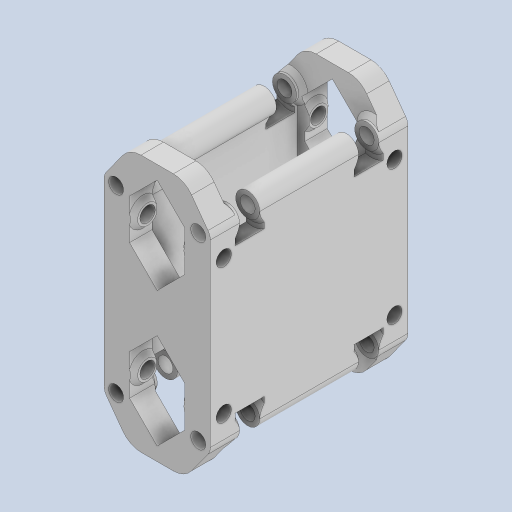
# Autodesk Inventor part: 3d_slider
Saved by Autodesk Inventor 2024 (Build 280153000, 153)
## iProperties
Created: 2023-08-10
Part Number: 3d_slider
Material: 一般
Document SubType Name: Modeling
Designer: zegi
Density: 1 g/cm^3
Appearance: 既定
Author: zegi
Autodesk Inventor part; units mm, degrees
ref_plane "YZ Plane" through (0, 0, 0) normal (1, 0, 0) x (0, 1, 0)
ref_plane "XZ Plane" through (0, 0, 0) normal (0, 1, 0) x (-1, 0, 0)
ref_plane "XY Plane" through (0, 0, 0) normal (0, 0, 1) x (1, 0, 0)
sketch "スケッチ1" plane through (0, 0, 0) normal (0, 0, 1) x (1, 0, 0)
  line L0 (-5.15, -39.6311) -> (5.15, -39.6311)
  line L1 (5.15, -39.6311) -> (5.15, 39.6311)
  line L2 (5.15, 39.6311) -> (-5.15, 39.6311)
  line L3 (-5.15, 39.6311) -> (-5.15, -39.6311)
  line L4 (-5.15, -39.6311) -> (5.15, 39.6311) construction
  line L5 (5.15, -39.6311) -> (-5.15, 39.6311) construction
  circle A0 centre (9.15, 20) radius 4 construction
  circle A1 centre (9.15, 20) radius 1.675
  circle A2 centre (9.15, 20) radius 2.675
  line L6 (9.15, 20) -> (9.15, 22.675) construction
  line L7 (6.475, 20) -> (11.825, 20) construction
  line L8 (9.15, 22.675) -> (0, 22.675)
  line L9 (0, 0) -> (0, 22.675)
  line L10 (11.825, 20) -> (11.825, 0)
  line L11 (11.825, 0) -> (0, 0)
  line L12 (7.825, 0) -> (7.825, 17.6762)
  circle A3 centre (9.15, 20) radius 4.675
  line L13 (0, 10.5) -> (6.15, 10.5)
  line L14 (6.15, 10.5) -> (6.15, 19.5)
  line L15 (6.15, 19.5) -> (0, 19.5)
  line L16 (0, 19.5) -> (0, 10.5)
  line L17 (0, 13.5) -> (6.15, 13.5) construction
  line L18 (6.15, 13.5) -> (6.15, 16.5)
  line L19 (6.15, 16.5) -> (0, 16.5) construction
  line L20 (0, 16.5) -> (0, 13.5)
  line L21 (6.15, 19.5) -> (0, 25.65)
  line L22 (6.15, 19.5) -> (14.8474, 19.5) construction
  line L23 (0, 19.5) -> (0, 28.65)
  line L24 (0, 28.65) -> (6.15, 28.65)
  line L25 (6.15, 28.65) -> (11.3109, 21.5767)
  line L26 (6.15, 10.5) -> (0, 4.35)
  line L27 (6.15, 10.5) -> (14.8474, 10.5) construction
  line L28 (7.825, 17.5422) -> (7.237, 18.1302)
  line L29 (7.825, 17.5422) -> (8.6565, 17.5422) construction
  point P0 (11.825, 16.1659)
  point P1 (7.825, 15.5167)
  point P2 (0, 15)
  point P3 (6.15, 15)
  point P4 (0, 19.5)
  point P5 (7.2802, 18.087)
  dimension "d0" = 10.3
  dimension "d2" = 8
  dimension "d3" = 3.35
  dimension "d4" = 1
  dimension "d5" = 20
  dimension "d6" = 4
  dimension "d14" = 2
  dimension "d23" = 9
  dimension "d24" = 15
  dimension "d25" = 3
  dimension "d31" = 1
  dimension "d46" = 135
  dimension "d47" = 3
  dimension "d48" = 135
  dimension "d50" = 135
  constraints: 60 end point, 8 perpendicular, 7 parallel, 6 horizontal, 6 midpoint, 6 point on circle, 6 point on line, 4 centre point, 3 equal length, 3 tangent, 2 vertical alignment, 1 coincident, 1 horizontal alignment, 1 vertical
  measures "d0" distance of L2.end L1.end
  measures "d2" diameter of A0
  measures "d3" diameter of A1
  measures "d4" radial gap between concentric circles of A1 A2
  measures "d5" vertical distance of L9.start A0.centre
  measures "d6" distance between parallel lines of L12 L10
  measures "d14" radial gap between concentric circles of A2 A3
  measures "d23" distance of L14.end L13.end
  measures "d24" distance from line of L11 point (0, 15)
  measures "d25" distance of L18.end L17.end
  measures "d31" distance between parallel lines of L14 L1
  measures "d46" angle of L22 L21
  measures "d47" distance from line of L24 L21.end
  measures "d48" angle of L26 L27
  measures "d50" angle of L29 L28
extrude "押し出し1" add sketch "スケッチ1" along normal blind 10 contours L12 A3 L10 L11 | A2 | L12 A2 L10 A3 | L28 A2 L12
extrude "押し出し2" add sketch "スケッチ1" along normal blind 1 from surface at 10 contours A2
extrude "押し出し4" add sketch "スケッチ1" along normal blind 6.5 from surface at 10 contours L12 A3 L10 L11
extrude "押し出し5" add sketch "スケッチ1" along normal blind 5.5 from surface at 16.5 contours L12 A3 L10 L11 | A2 | L12 A2 L10 A3
extrude "押し出し6" add sketch "スケッチ1" against normal blind 1 from surface at 16.5 contours A2
sketch "スケッチ2" plane through (11.825, 0, 0) normal (1, 0, 0) x (0, 0, -1)
  line L0 (-16.5, 20) -> (-22, 20) projected
  line L1 (-22, 20) -> (-22, 0) projected
  line L2 (0, 0) -> (-22, 0) projected
  line L3 (0, 0) -> (0, 20) projected
  line L4 (0, 20) -> (-10, 20) projected
  line L5 (-10, 16.1659) -> (-10, 20) projected
  line L6 (-16.5, 20) -> (-16.5, 16.1659) projected
  line L7 (-22, 15) -> (0, 15)
  circle A0 centre (-19, 15) radius 4 construction
  line L8 (15, -35.6596) -> (-15, -35.6596)
  line L9 (-15, -35.6596) -> (-15, 35.6596)
  line L10 (-15, 35.6596) -> (15, 35.6596)
  line L11 (15, 35.6596) -> (15, -35.6596)
  line L12 (15, -35.6596) -> (-15, 35.6596) construction
  line L13 (-15, -35.6596) -> (15, 35.6596) construction
  line L14 (-10, 16.1659) -> (-16.5, 16.1659) projected
  point P0 (0, 0)
  point P1 (-11, 0)
  point P2 (-11, 15)
  dimension "d26" = 15
  dimension "d27" = 8
  dimension "d28" = 30
  constraints: 14 end point, 4 midpoint, 3 point on line, 2 parallel, 2 perpendicular, 1 centre point, 1 coincident, 1 horizontal, 1 tangent
  measures "d26" distance of point (-11, 0) point (-11, 15)
  measures "d27" diameter of A0
  measures "d28" distance of L9.end L10.end
extrude "押し出し7" add sketch "スケッチ1" against normal blind 5 from surface at 22 contours L11 L9 L26 L1 | L1 L26 L14 A3 L12 L11 | L12 A3 L10 L11 | L24 L25 A3 L8 L1 | L1 L8 L21 L23 L24 | A2 | A3 L14 L21 L1 L8 A2 L28 L12 | L12 A2 L10 A3 | L8 A3 L1 | L1 A3 L21 L8 | L28 A2 L12 | L1 L21 A3 | A3 L25 A2 L8
hole "穴1" at (11.825, 15, 19) direction (-1, 0, 0) diameter 3.4 end through all
sketch "スケッチ3" plane through (6.15, 10.5, 22) normal (-1, 0, 0) x (0, 0, 1)
  circle A0 centre (-3, 4.5) radius 1.7 projected
  circle A1 centre (-3, 4.5) radius 2.2
  line L0 (-5, 0) -> (-5, 9) projected
  point P0 (-22, -10.5)
  point P1 (-5, 5.4165)
  point P2 (-5, 3.5835)
  dimension "d40" = 0.5
  constraints: 1 centre point
  measures "d40" radial gap between concentric circles of A0 A1
extrude "押し出し8" add sketch "スケッチ3" along normal blind 1 contours A1 L0 picked at (-4.9, 4.5)
chamfer "面取り1" distance 1 angle 45 1 edges at (6.15, 15, 21.2)
fillet "フィレット3" radius 5 1 edges at (6.15, 28.65, 19.5)
chamfer "面取り2" distance 1 angle 45 3 edges at (10.1878, 17.5345, 10) (10.4937, 17.687, 16.5) (7.1555, 21.7825, 17)
mirror "ミラー7" about plane through (0, 25.65, 0) normal (-1, 0, 0)
mirror "ミラー8" about plane through (9.15, 11.3375, 0) normal (0, 0, -1)
mirror "ミラー9" about plane through (7.825, 0, 0) normal (0, -1, 0)
